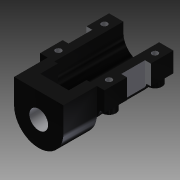
# Autodesk Inventor part: CueHolderBottom
Saved by Autodesk Inventor 2015 (Build 190159000, 159)
## iProperties
Created: 2017-01-09
Part Number: CueHolderBottom
Material: Generic
Document SubType Name: Modeling
Designer: Ernest
Density: 1 g/cm^3
Appearance: Default
Mass: 9.52114 g
Surface Area: 51.2118 cm^2
Volume: 9.52114 cm^3
Author: Ernest
Autodesk Inventor part; units mm, degrees
ref_plane "YZ Plane" through (0, 0, 0) normal (1, 0, 0) x (0, 1, 0)
ref_plane "XZ Plane" through (0, 0, 0) normal (0, 1, 0) x (-1, 0, 0)
ref_plane "XY Plane" through (0, 0, 0) normal (0, 0, 1) x (1, 0, 0)
sketch "Sketch1" plane through (0, 0, 0) normal (0, 0, 1) x (1, 0, 0)
  circle A0 centre (0, 0) radius 3
  circle A1 centre (51.029, 0) radius 3
  circle A2 centre (0, 0) radius 6
  circle A3 centre (51.029, 0) radius 6
  line L0 (11.2237, 0) -> (17.9507, 0)
  line L1 (33.0783, 0) -> (39.8053, 0)
  line L2 (16.4475, -5) -> (16.4475, 0)
  line L3 (34.5815, -5) -> (34.5815, 0)
  line L4 (18.5272, 44.067) -> (39.0012, 44.067) construction
  line L5 (8.015, 33.5) -> (43.014, 33.5) construction
  line L6 (43.014, 33.5) -> (43.014, 15.5) construction
  line L7 (43.014, 15.5) -> (8.015, 15.5) construction
  line L8 (8.015, 15.5) -> (8.015, 33.5) construction
  line L9 (14.489, 24.5) -> (38.452, 24.5) construction
  line L10 (22.5145, 29) -> (28.5145, 29)
  line L11 (28.5145, 29) -> (28.5145, 20)
  line L12 (28.5145, 20) -> (22.5145, 20)
  line L13 (22.5145, 20) -> (22.5145, 29)
  line L14 (25.5145, 33.5) -> (25.5145, 15.5) construction
  line L15 (4.5826, 10) -> (46.4464, 10)
  line L16 (-13, 10) -> (-13, -10)
  line L17 (64.029, 10) -> (64.029, -10)
  line L18 (-13, 10) -> (-4.5826, 10)
  line L19 (-13, -10) -> (-4.5826, -10)
  line L20 (64.029, 10) -> (55.6116, 10)
  line L21 (64.029, -10) -> (55.6116, -10)
  arc A4 (11.8571, -10) -> (39.1719, -10) centre (25.5145, -5) ccw
  arc A5 (16.4475, -5) -> (34.5815, -5) centre (25.5145, -5) ccw
  arc A6 (33.0783, 0) -> (17.9507, 0) centre (25.5145, -5) ccw
  line L22 (46.4464, -10) -> (39.1719, -10)
  line L23 (4.5826, -10) -> (11.8571, -10)
  line L24 (11.2237, 0) -> (11.2237, -10)
  line L25 (39.8053, 0) -> (39.8053, -10)
  arc A7 (46.4464, -10) -> (55.6116, -10) centre (51.029, 0) ccw
  arc A8 (55.6116, 10) -> (46.4464, 10) centre (51.029, 0) ccw
  arc A9 (4.5826, 10) -> (-4.5826, 10) centre (0, 0) ccw
  arc A10 (-4.5826, -10) -> (4.5826, -10) centre (0, 0) ccw
  line L26 (30.5145, 26.5) -> (17.5145, 26.5)
  line L27 (17.5145, 26.5) -> (17.5145, 10)
  line L28 (17.5145, 10) -> (30.5145, 10)
  line L29 (30.5145, 10) -> (30.5145, 26.5)
  line L30 (-13, 0) -> (64.029, 0)
  point P0 (6, 0)
  point P1 (45.029, 0)
  dimension "d144" = 12
  dimension "d146" = 12
  dimension "d143" = 6
  dimension "d145" = 6
  dimension "d147" = 51.029
  dimension "d148" = 77.029
  dimension "d149" = 20
  dimension "d150" = 11
  dimension "d151" = 11
  dimension "d152" = 11
  dimension "d153" = 11
  dimension "d154" = 9.067
  dimension "d155" = 25.5145
  dimension "d156" = 5
  dimension "d157" = 9.067
  dimension "d158" = 13
  dimension "d159" = 14.5439
  dimension "d160" = 11.2238
  dimension "d161" = 11.2238
  constraints: 62 end point, 14 point on circle, 11 point on line, 9 centre point, 9 horizontal, 7 parallel, 7 perpendicular, 6 coincident, 6 midpoint, 5 collinear, 2 horizontal alignment, 2 tangent, 2 vertical, 4 other
  measures "d143" diameter of A0
  measures "d145" diameter of A1
  measures "d147" distance of A1.centre point (0, 0)
  measures "d148" distance of L30.end L30.start
  measures "d149" distance between parallel lines of L18 L19
  measures "d150" radius of A9
  measures "d151" radius of A10
  measures "d152" radius of A8
  measures "d153" radius of A7
  measures "d154" radius of A6
  measures "d155" horizontal distance of point (0, 0) A5.centre
  measures "d156" vertical distance of point (0, 0) A5.centre
  measures "d157" radius of A5
  measures "d158" distance from line of point (0, 0) L16
  measures "d159" radius of A4
  measures "d160" distance from line of point (0, 0) L24
  measures "d161" distance from line of A1.centre L25
extrude "Extrusion1" add sketch "Sketch1" along normal blind 35 contours L30 A0 | L30 A2 A0 | A0 L30 A2 | A0 L30 | L30 L24 L23 A10 L19 L16 A2 | A2 L30 L16 L18 A9 L15 A8 L20 L17 A3 L1 A6 L0 | L0 L2 A5 L3 L1 L25 L22 A4 L23 L24 | L0 L30 L1 L3 A5 L2 | A6 L30 | L25 L30 A3 L17 L21 A7 L22 | L27 L26 L13 L12 L11 L29 L15 | L30 A1 A3 | A3 L30 A1 | L26 L11 L12 L13 | L30 A1 | A1 L30
extrude "Extrusion2" cut sketch "Sketch1" along normal blind 35 contours L30 A0 | L30 A2 A0 | A0 L30 A2 | A0 L30 | L0 L30 L1 L3 A5 L2 | A6 L30 | L30 A1 A3 | A3 L30 A1 | L30 A1 | A1 L30
ref_plane "Work Plane1" through (55.6116, 0, 0) normal (0, 1, 0) x (1, 0, 0)
sketch "Sketch2" plane through (55.6116, 0, 0) normal (0, 1, 0) x (1, 0, 0)
  line L0 (-61.6116, -35) -> (-61.6116, 0)
  line L1 (-68.6116, 0) -> (-61.6116, 0)
  line L2 (-68.6116, -35) -> (-68.6116, 0)
  line L3 (-68.6116, -35) -> (-61.6116, -35)
  line L4 (1.4174, 0) -> (1.4174, -35)
  line L5 (1.4174, -35) -> (8.4174, -35)
  line L6 (8.4174, -35) -> (8.4174, 0)
  line L7 (1.4174, 0) -> (8.4174, 0)
  line L8 (-60.0873, -35) -> (-68.6116, -35)
  line L9 (-68.6116, 0) -> (-67.4686, 0)
  line L10 (-67.4686, 0) -> (-67.4686, -35)
  line L11 (-67.4686, -35) -> (-68.6116, -35)
  line L12 (-68.6116, -35) -> (-68.6116, 0)
  line L13 (1.4174, -35) -> (8.4174, -35)
  line L14 (8.4174, 0) -> (7.2744, 0)
  line L15 (7.2744, 0) -> (7.2744, -35)
  line L16 (7.2744, -35) -> (8.4174, -35)
  line L17 (8.4174, -35) -> (8.4174, 0)
  circle A0 centre (-64.5401, -17.5) radius 1.5
  circle A1 centre (4.3459, -17.5) radius 1.5
  circle A2 centre (-46.6831, -17.5) radius 1.5
  circle A3 centre (-13.5111, -17.5) radius 1.5
  line L18 (-49.6116, 0) -> (-49.6116, -35)
  line L19 (-49.6116, -35) -> (-37.6608, -35)
  line L20 (-37.6608, -35) -> (-37.6608, 0)
  line L21 (-49.6116, 0) -> (-37.6608, 0)
  line L22 (-10.5826, -35) -> (-10.5826, 0)
  line L23 (-22.5333, 0) -> (-10.5826, 0)
  line L24 (-22.5333, -35) -> (-22.5333, 0)
  line L25 (-22.5333, -35) -> (-10.5826, -35)
  circle A4 centre (-42.9266, -5.833) radius 1.5
  circle A5 centre (-42.9266, -29.167) radius 1.5
  circle A6 centre (-17.2676, -5.833) radius 1.5
  circle A7 centre (-17.2676, -29.167) radius 1.5
  line L26 (1.4174, -0.0847) -> (1.4174, -35.0847)
  line L27 (-49.6116, -0.0847) -> (-49.6116, -35.0847)
  line L28 (-49.6116, -35) -> (-61.6116, -35) projected
  line L29 (-61.6116, 0) -> (-49.6116, 0) projected
  line L30 (1.4174, -35) -> (-10.5826, -35) projected
  line L31 (-10.5826, 0) -> (1.4174, 0) projected
  line L32 (-68.6116, 0) -> (-68.6116, -35) projected
  line L33 (-68.6116, 0) -> (-68.6116, -35) projected
  line L34 (-10.5826, 0) -> (1.4174, 0) projected
  line L35 (-61.6116, 0) -> (-49.6116, 0) projected
  line L36 (-25.0971, 0) -> (-38.0971, 0) projected
  line L37 (-9.1652, 0) -> (-25.0971, 0) projected
  line L38 (0, 0) -> (-9.1652, 0) projected
  line L39 (8.4174, 0) -> (0, 0) projected
  line L40 (0, 0) -> (8.4174, 0) projected
  line L41 (-9.1652, 0) -> (0, 0) projected
  line L42 (-16.4396, 0) -> (-9.1652, 0) projected
  line L43 (-43.7545, 0) -> (-16.4396, 0) projected
  line L44 (-51.029, 0) -> (-43.7545, 0) projected
  line L45 (-60.1942, 0) -> (-51.029, 0) projected
  line L46 (-68.6116, 0) -> (-60.1942, 0) projected
  line L47 (-60.1942, 0) -> (-68.6116, 0) projected
  line L48 (-51.029, 0) -> (-60.1942, 0) projected
  line L49 (-38.0971, 0) -> (-51.029, 0) projected
  line L50 (8.4174, 0) -> (8.4174, -35) projected
  line L51 (8.4174, 0) -> (8.4174, -35) projected
  line L52 (1.4174, -35) -> (-10.5826, -35) projected
  line L53 (-49.6116, -35) -> (-61.6116, -35) projected
  line L54 (-16.4396, -35) -> (-9.1652, -35) projected
  line L55 (-9.1652, -35) -> (0, -35) projected
  line L56 (0, -35) -> (8.4174, -35) projected
  line L57 (8.4174, -35) -> (0, -35) projected
  line L58 (0, -35) -> (-9.1652, -35) projected
  line L59 (-9.1652, -35) -> (-25.0971, -35) projected
  line L60 (-25.0971, -35) -> (-38.0971, -35) projected
  line L61 (-38.0971, -35) -> (-51.029, -35) projected
  line L62 (-51.029, -35) -> (-60.1942, -35) projected
  line L63 (-60.1942, -35) -> (-68.6116, -35) projected
  line L64 (-68.6116, -35) -> (-60.1942, -35) projected
  line L65 (-60.1942, -35) -> (-51.029, -35) projected
  line L66 (-51.029, -35) -> (-43.7545, -35) projected
  line L67 (-43.7545, -35) -> (-16.4396, -35) projected
  line L68 (-68.6116, 0) -> (8.4174, 0)
  line L69 (8.4174, 0) -> (8.4174, -35)
  line L70 (8.4174, -35) -> (-68.6116, -35)
  line L71 (-68.6116, -35) -> (-68.6116, 0)
  point P0 (-55.5011, -35.0847)
  dimension "d50" = 3
  dimension "d52" = 3
  dimension "d58" = 35
  dimension "d59" = 17.5
  dimension "d60" = 17.5
  dimension "d61" = 3
  dimension "d62" = 3
  dimension "d63" = 17.5
  dimension "d64" = 17.5
  dimension "d65" = 2.9285
  dimension "d66" = 2.9285
  dimension "d67" = 3
  dimension "d68" = 3
  dimension "d69" = 3
  dimension "d70" = 3
  dimension "d71" = 5.833
  dimension "d72" = 5.833
  dimension "d73" = 5.833
  dimension "d74" = 5.833
  dimension "d75" = 6.685
  dimension "d76" = 6.685
  dimension "d77" = 6.685
  dimension "d78" = 6.685
  dimension "d139" = 5.857
  dimension "d140" = 5.857
  dimension "d141" = 2.9285
  dimension "d142" = 2.9285
  dimension "d166" = 1.143
  dimension "d168" = 12
  dimension "d169" = 12
  dimension "d170" = 15.1275
  dimension "d171" = 11.9507
  dimension "d172" = 11.9507
  dimension "d173" = 1.143
  constraints: 64 end point, 15 collinear, 8 centre point, 6 parallel, 3 horizontal, 3 perpendicular, 2 point on line
  measures "d50" diameter of A0
  measures "d52" diameter of A1
  measures "d58" distance of L0.start L0.end
  measures "d59" distance from line of L8 A0.centre
  measures "d60" distance from line of L5 A1.centre
  measures "d61" diameter of A2
  measures "d62" diameter of A3
  measures "d63" distance from line of L8 A2.centre
  measures "d64" distance from line of L13 A3.centre
  measures "d65" distance from line of L18 A2.centre
  measures "d66" distance from line of L22 A3.centre
  measures "d67" diameter of A4
  measures "d68" diameter of A5
  measures "d69" diameter of A6
  measures "d70" diameter of A7
  measures "d71" distance from line of L21 A4.centre
  measures "d72" distance from line of L19 A5.centre
  measures "d73" distance from line of L23 A6.centre
  measures "d74" distance from line of L25 A7.centre
  measures "d75" distance from line of L18 A4.centre
  measures "d76" distance from line of L18 A5.centre
  measures "d77" distance from line of L22 A6.centre
  measures "d78" distance from line of L22 A7.centre
  measures "d139" distance between parallel lines of L0 L10
  measures "d140" distance between parallel lines of L15 L4
  measures "d141" distance from line of L0 A0.centre
  measures "d142" distance from line of L4 A1.centre
  measures "d166" distance between parallel lines of L15 L17
  measures "d168" distance between parallel lines of L18 L0
  measures "d169" distance between parallel lines of L26 L22
  measures "d170" distance between parallel lines of L24 L20
  measures "d171" distance of L18.start L20.end
  measures "d172" distance of L23.start L22.end
  measures "d173" distance between parallel lines of L2 L10
extrude "Extrusion3" cut sketch "Sketch2" along normal mid plane 35 contours L3 L2 L1 L10 | L7 L6 L5 L15 | A0 | A1 | A2 | A3 | A4 | A5 | A6 | A7
sketch "Sketch3" plane through (30.5145, 10, 0) normal (1, 0, 0) x (0, 0, -1)
  line L0 (-35, 0) -> (-35, 16.5) projected
  line L1 (-35, 14.5) -> (0, 14.5) construction
  line L2 (0, 0) -> (0, 16.5) projected
  line L3 (0, 0) -> (0, 16.5) projected
  line L4 (0, 16.5) -> (-35, 16.5) projected
  line L5 (-35, 0) -> (-35, 16.5) projected
  line L6 (0, 0) -> (-35, 0) projected
  line L7 (-35, 19) -> (0, 19)
  line L8 (0, 19) -> (0, 10)
  line L9 (0, 10) -> (-35, 10)
  line L10 (-35, 10) -> (-35, 19)
  line L11 (-35, 10) -> (0, 10)
  line L12 (0, 10) -> (0, 8.4)
  line L13 (-32.5098, 8.4) -> (-34.5098, 8.4)
  line L14 (-35, 8.4) -> (-35, 10)
  arc A0 (-35, 9.054) -> (-35, 9.746) centre (-34.5098, 9.4) ccw
  circle A1 centre (-32.5098, 9.4) radius 0.6
  line L15 (-33.7098, 9.2) -> (-33.3098, 9.2)
  arc A2 (-33.9098, 9.4) -> (-33.7098, 9.2) centre (-33.7098, 9.4) ccw
  arc A3 (-33.3098, 9.2) -> (-33.1098, 9.4) centre (-33.3098, 9.4) ccw
  arc A4 (-35, 9.746) -> (-35, 9.054) centre (-34.5098, 9.4) ccw
  line L16 (-34.5098, 8.8) -> (-34.5098, 8.4)
  line L17 (-32.5098, 8.8) -> (-32.5098, 8.4)
  point P0 (0, -10)
  point P1 (-35, 9.2)
  point P2 (0, 9.2)
  point P3 (-33.9098, 9.4)
  point P4 (-33.1098, 9.4)
  dimension "d83" = 2
  dimension "d84" = 9
  dimension "d85" = 4.5
  dimension "d86" = 1.6
  dimension "d87" = 1.2
  dimension "d88" = 1.2
  dimension "d89" = 2
  dimension "d90" = 0.8
  dimension "d91" = 0.2
  constraints: 24 end point, 12 point on circle, 8 point on line, 5 centre point, 5 horizontal, 5 perpendicular, 4 parallel, 4 tangent, 2 coincident, 2 midpoint, 1 equal radius, 8 other
  measures "d83" distance between parallel lines of L1 L4
  measures "d84" distance between parallel lines of L9 L7
  measures "d85" distance between parallel lines of L1 L7
  measures "d86" distance between parallel lines of L11 L13
  measures "d87" diameter of A0
  measures "d88" diameter of A1
  measures "d89" distance of A1.centre A0.centre
  measures "d90" distance between parallel lines of L15 L13
  measures "d91" radius of A2
extrude "Extrusion4" cut sketch "Sketch3" against normal blind 7 contours L0 A0 | A0 A2 L15 A3 A1 L17 L13 L16 | A1
pattern_linear "Rectangular Pattern1" count 18 spacing 2 along (0, 0, -1) count 2 spacing 2 along (0, 0, 1) of "Extrusion4"
sketch "Sketch4" plane through (0, 0, 35) normal (0, 0, 1) x (1, 0, 0)
  line L0 (23.5145, 18.4) -> (23.5145, 19.746) projected
  line L1 (23.5145, 19.746) -> (30.5145, 19.746) projected
  line L2 (30.5145, 19.746) -> (30.5145, 26.5) projected
  line L3 (30.5145, 26.5) -> (17.5145, 26.5) projected
  line L4 (17.5145, 26.5) -> (17.5145, 10) projected
  line L5 (17.5145, 10) -> (4.5826, 10) projected
  arc A0 (4.5826, 10) -> (-4.5826, 10) centre (0, 0) ccw projected
  line L6 (-4.5826, 10) -> (-13, 10) projected
  line L7 (64.029, 10) -> (55.6116, 10) projected
  arc A1 (55.6116, 10) -> (46.4464, 10) centre (51.029, 0) ccw projected
  line L8 (46.4464, 10) -> (30.5145, 10) projected
  line L9 (30.5145, 10) -> (30.5145, 18.4) projected
  line L10 (30.5145, 18.4) -> (23.5145, 18.4) projected
  line L11 (17.5145, 10) -> (12.5145, 10)
  line L12 (12.5145, 10) -> (12.5145, 18)
  line L13 (12.5145, 18) -> (17.5145, 18)
  line L14 (17.5145, 18) -> (17.5145, 10)
  line L15 (30.5145, 10) -> (35.5145, 10)
  line L16 (35.5145, 10) -> (35.5145, 18)
  line L17 (35.5145, 18) -> (30.5145, 18)
  line L18 (30.5145, 18) -> (30.5145, 10)
  circle A2 centre (0, 0) radius 6 projected
  circle A3 centre (51.029, 0) radius 6 projected
  line L19 (-13, -10) -> (-4.5826, -10) projected
  arc A4 (-4.5826, -10) -> (4.5826, -10) centre (0, 0) ccw projected
  line L20 (4.5826, -10) -> (11.8571, -10) projected
  arc A5 (11.8571, -10) -> (39.1719, -10) centre (25.5145, -5) ccw projected
  line L21 (39.1719, -10) -> (46.4464, -10) projected
  arc A6 (46.4464, -10) -> (55.6116, -10) centre (51.029, 0) ccw projected
  line L22 (55.6116, -10) -> (64.029, -10) projected
  line L23 (-13, 10) -> (-13, -10) projected
  line L24 (64.029, -10) -> (64.029, 10) projected
  dimension "d100" = 8
  dimension "d101" = 5
  dimension "d106" = 5
  dimension "d107" = 8
  constraints: 16 end point, 4 parallel, 2 horizontal, 2 perpendicular
  measures "d100" distance of L11.end L12.end
  measures "d101" distance of L12.end L13.end
  measures "d106" distance of L17.end L16.end
  measures "d107" distance of L16.end L15.end
extrude "Extrusion5" add sketch "Sketch4" against normal blind 26.25 contours L17 L16 L8 L9 | L4 L5 L12 L13
extrude "Extrusion6" cut sketch "Sketch4" against normal blind 8.75 contours L17 L16 L8 L9 | L4 L5 L12 L13
sketch "Sketch5" plane through (17.5145, 26.5, 0) normal (0, 1, 0) x (1, 0, 0)
  arc A0 (0, -26.25) -> (0, -23.75) centre (0, -25) ccw
  line L0 (-5, -26.25) -> (0, -26.25) projected
  line L1 (-5, -8.75) -> (0, -8.75) projected
  arc A1 (0, -21.25) -> (0, -23.75) centre (0, -22.5) ccw
  arc A2 (0, -21.25) -> (0, -18.75) centre (0, -20) ccw
  arc A3 (0, -16.25) -> (0, -18.75) centre (0, -17.5) ccw
  arc A4 (0, -16.25) -> (0, -13.75) centre (0, -15) ccw
  arc A5 (0, -11.25) -> (0, -13.75) centre (0, -12.5) ccw
  arc A6 (0, -11.25) -> (0, -8.75) centre (0, -10) ccw
  arc A7 (13, -23.75) -> (13, -26.25) centre (13, -25) ccw
  line L2 (13, -26.25) -> (18, -26.25) projected
  arc A8 (13, -23.75) -> (13, -21.25) centre (13, -22.5) ccw
  arc A9 (13, -18.75) -> (13, -21.25) centre (13, -20) ccw
  arc A10 (13, -18.75) -> (13, -16.25) centre (13, -17.5) ccw
  arc A11 (13, -13.75) -> (13, -16.25) centre (13, -15) ccw
  arc A12 (13, -13.75) -> (13, -11.25) centre (13, -12.5) ccw
  arc A13 (13, -8.75) -> (13, -11.25) centre (13, -10) ccw
  line L3 (-29.291, -35) -> (0, -35)
  line L4 (0, 0) -> (-29.291, 0)
  line L5 (-29.291, 0) -> (-29.291, -35)
  line L6 (45.3715, -35) -> (13, -35)
  line L7 (13, 0) -> (45.3715, 0)
  line L8 (45.3715, 0) -> (45.3715, -35)
  line L9 (-5, -26.25) -> (0, -26.25)
  line L10 (0, -8.75) -> (-5, -8.75)
  line L11 (-5, -8.75) -> (-5, -26.25)
  line L12 (18, -26.25) -> (13, -26.25)
  line L13 (13, -8.75) -> (18, -8.75)
  line L14 (18, -8.75) -> (18, -26.25)
  line L15 (0, -8.75) -> (0, 0)
  line L16 (0, -35) -> (0, -26.25)
  line L17 (13, -35) -> (13, -26.25)
  line L18 (13, -8.75) -> (13, 0)
  line L19 (0, -35) -> (13, -35)
  line L20 (0, 0) -> (13, 0)
  dimension "d108" = 2.5
  dimension "d109" = 17.5
  dimension "d110" = 2.5
  dimension "d111" = 2.5
  dimension "d112" = 2.5
  dimension "d113" = 2.5
  dimension "d114" = 2.5
  dimension "d115" = 2.5
  dimension "d116" = 2.5
  dimension "d117" = 2.5
  dimension "d118" = 2.5
  dimension "d119" = 2.5
  dimension "d120" = 2.5
  dimension "d121" = 2.5
  dimension "d122" = 2.5
  dimension "d162" = 5
  dimension "d163" = 5
  dimension "d164" = 13
  dimension "d165" = 74.6625
  constraints: 37 end point, 28 point on circle, 14 centre point, 13 tangent, 6 equal length, 5 horizontal, 1 point on line
  measures "d108" diameter of A0
  measures "d109" distance between parallel lines of L1 L0
  measures "d110" diameter of A1
  measures "d111" diameter of A2
  measures "d112" diameter of A3
  measures "d113" diameter of A4
  measures "d114" diameter of A5
  measures "d115" diameter of A6
  measures "d116" diameter of A7
  measures "d117" diameter of A8
  measures "d118" diameter of A9
  measures "d119" diameter of A10
  measures "d120" diameter of A11
  measures "d121" diameter of A12
  measures "d122" diameter of A13
  measures "d162" distance between parallel lines of L16 L11
  measures "d163" distance between parallel lines of L17 L14
  measures "d164" distance between parallel lines of L18 L15
  measures "d165" distance between parallel lines of L8 L5
extrude "Extrusion7" cut sketch "Sketch5" against normal blind 16.5 contours A0 A1 A2 A3 A4 A5 A6 L15 L20 L18 A13 A12 A11 A10 A9 A8 A7 L17 L19 L16
sketch "Sketch6" plane through (17.5145, 26.5, 25) normal (0, 1, 0) x (1, 0, 0)
  line L0 (-2.8394, -2.9296) -> (15.1567, -2.9296)
  line L1 (15.1567, -2.9296) -> (15.1567, 18.0113)
  line L2 (15.1567, 18.0113) -> (-2.8394, 18.0113)
  line L3 (-2.8394, 18.0113) -> (-2.8394, -2.9296)
  point P0 (-17.5145, 25)
  constraints: 8 end point, 2 parallel, 1 horizontal, 1 perpendicular
extrude "Extrusion8" cut sketch "Sketch6" against normal blind 8.5
sketch "Sketch7" plane through (35.5145, 10, 8.75) normal (1, 0, 0) x (0, 0, -1)
  line L0 (-17.5, 8) -> (-17.5, 0) projected
  line L1 (0, 0) -> (-17.5, 0) projected
  line L2 (0, 8) -> (0, 0) projected
  line L3 (-17.5, 8) -> (0, 8) projected
  line L4 (-10.25, 0) -> (-7.25, 0) projected
  line L5 (1.417, 0) -> (4.417, 0) projected
  circle A0 centre (-13.125, 4) radius 1.5
  circle A1 centre (-4.375, 4) radius 1.5
  line L6 (-8.75, 8) -> (-8.75, 0)
  line L7 (-17.5, 0) -> (0, 0) projected
  point P0 (8.75, -10)
  point P1 (-7.25, -10)
  point P2 (-10.25, -10)
  point P3 (-18.917, -10)
  point P4 (-21.917, -10)
  dimension "d127" = 3
  dimension "d128" = 3
  dimension "d129" = 8
  dimension "d130" = 17.5
  dimension "d131" = 8.75
  dimension "d132" = 4
  dimension "d133" = 4
  dimension "d134" = 4.375
  dimension "d135" = 4.375
  constraints: 2 centre point, 2 end point, 2 midpoint, 1 vertical
  measures "d127" diameter of A0
  measures "d128" diameter of A1
  measures "d129" distance of L0.start L0.end
  measures "d130" distance of L0.start L2.start
  measures "d131" distance between parallel lines of L0 L6
  measures "d132" distance from line of L3 A0.centre
  measures "d133" distance from line of L1 A1.centre
  measures "d134" distance from line of L0 A0.centre
  measures "d135" distance from line of L2 A1.centre
extrude "Extrusion9" cut sketch "Sketch7" against normal blind 25.75 contours A0 | A1
sketch "Sketch8" plane through (39.1719, -10, 0) normal (0, -1, 0) x (1, 0, 0)
  spline S0 degree 5 poles (0, 4.5822) (-0.1104, 4.5091) (-0.2304, 4.4472) (-0.3605, 4.3972) (-0.5007, 4.3614) (-0.796, 4.3262) (-0.9501, 4.3258) (-1.1137, 4.3457) (-1.2845, 4.3916) (-1.5743, 4.5255) (-1.6926, 4.5954) (-1.8098, 4.6839) (-1.9216, 4.7931) (-2.1281, 5.0647) (-2.2209, 5.2289) (-2.2923, 5.4191) (-2.3279, 5.6262) (-2.3279, 5.996) (-2.3055, 6.1592) (-2.2618, 6.314) (-2.2005, 6.4555) (-2.0783, 6.6675) (-2.0237, 6.746) (-1.965, 6.8175) (-1.9034, 6.8822) (-1.7429, 7.0289) (-1.6416, 7.102) (-1.5389, 7.1611) (-1.4367, 7.2081) (-1.0141, 7.3602) (-0.7042, 7.3683) (-0.4373, 7.3138) (-0.2033, 7.2184) (0, 7.0838) knots 0 0 0 0 0 0 0.150257 0.150257 0.150257 0.150257 0.296295 0.296295 0.296295 0.296295 0.395447 0.395447 0.395447 0.395447 0.50046 0.50046 0.50046 0.50046 0.583231 0.583231 0.583231 0.583231 0.63924 0.63924 0.63924 0.63924 0.725202 0.725202 0.725202 0.725202 1 1 1 1 1 1 projected
  arc A0 (0, 4.5822) -> (0, 7.0838) centre (-0.8279, 5.833) ccw projected
  circle A1 centre (-0.8279, 5.833) radius 1.5 projected
  spline S1 degree 5 poles (0, 27.9162) (-0.1104, 27.8431) (-0.2304, 27.7812) (-0.3605, 27.7312) (-0.5007, 27.6954) (-0.796, 27.6602) (-0.9501, 27.6598) (-1.1137, 27.6797) (-1.2845, 27.7256) (-1.5743, 27.8595) (-1.6926, 27.9294) (-1.8098, 28.0179) (-1.9216, 28.1271) (-2.1281, 28.3987) (-2.2209, 28.5629) (-2.2923, 28.7531) (-2.3279, 28.9602) (-2.3279, 29.33) (-2.3055, 29.4932) (-2.2618, 29.648) (-2.2005, 29.7895) (-2.0783, 30.0015) (-2.0237, 30.08) (-1.965, 30.1515) (-1.9034, 30.2162) (-1.7429, 30.3629) (-1.6416, 30.436) (-1.5389, 30.4951) (-1.4367, 30.5421) (-1.0141, 30.6942) (-0.7042, 30.7023) (-0.4373, 30.6478) (-0.2033, 30.5524) (0, 30.4178) knots 0 0 0 0 0 0 0.150257 0.150257 0.150257 0.150257 0.296295 0.296295 0.296295 0.296295 0.395447 0.395447 0.395447 0.395447 0.50046 0.50046 0.50046 0.50046 0.583231 0.583231 0.583231 0.583231 0.63924 0.63924 0.63924 0.63924 0.725202 0.725202 0.725202 0.725202 1 1 1 1 1 1 projected
  arc A2 (0, 27.9162) -> (0, 30.4178) centre (-0.8279, 29.167) ccw projected
  circle A3 centre (-0.8279, 29.167) radius 1.5 projected
  spline S2 degree 8 poles (-27.3149, 30.4178) (-27.2459, 30.4635) (-27.1734, 30.5052) (-27.0975, 30.5428) (-27.018, 30.576) (-26.9349, 30.6044) (-26.8483, 30.6277) (-26.7581, 30.6453) (-26.5735, 30.6673) (-26.4794, 30.6721) (-26.3822, 30.6702) (-26.2818, 30.6609) (-26.1786, 30.6433) (-26.073, 30.6163) (-25.9657, 30.5785) (-25.7845, 30.4948) (-25.7108, 30.4553) (-25.6372, 30.4097) (-25.5641, 30.3575) (-25.4923, 30.2984) (-25.4225, 30.2318) (-25.3557, 30.1575) (-25.2689, 30.0433) (-25.2454, 30.0104) (-25.2226, 29.9763) (-25.2006, 29.9411) (-25.1794, 29.9047) (-25.1592, 29.8672) (-25.1401, 29.8287) (-25.0904, 29.7196) (-25.0387, 29.5867) (-25, 29.4439) (-24.9772, 29.294) (-24.9719, 29.1407) (-24.9851, 28.9871) (-25.0151, 28.8414) (-25.059, 28.703) (-25.0928, 28.6126) (-25.1046, 28.5832) (-25.117, 28.5543) (-25.13, 28.526) (-25.1436, 28.4981) (-25.1577, 28.4709) (-25.1722, 28.4442) (-25.2181, 28.3646) (-25.2508, 28.3136) (-25.2853, 28.2651) (-25.3211, 28.2191) (-25.3582, 28.1756) (-25.3963, 28.1346) (-25.4353, 28.0961) (-25.5355, 28.0044) (-25.5978, 27.9545) (-25.661, 27.9099) (-25.7247, 27.8703) (-25.7886, 27.8354) (-25.8524, 27.8048) (-25.9159, 27.7783) (-26.18, 27.6832) (-26.3771, 27.6493) (-26.564, 27.6458) (-26.7386, 27.6664) (-26.9004, 27.7061) (-27.0499, 27.762) (-27.1878, 27.8321) (-27.3149, 27.9162) knots 0 0 0 0 0 0 0 0 0 0.150381 0.150381 0.150381 0.150381 0.150381 0.150381 0.150381 0.29654 0.29654 0.29654 0.29654 0.29654 0.29654 0.29654 0.395774 0.395774 0.395774 0.395774 0.395774 0.395774 0.395774 0.433966 0.433966 0.433966 0.433966 0.433966 0.433966 0.433966 0.500813 0.556206 0.556206 0.556206 0.556206 0.556206 0.556206 0.556206 0.583535 0.583535 0.583535 0.583535 0.583535 0.583535 0.583535 0.639503 0.639503 0.639503 0.639503 0.639503 0.639503 0.639503 0.725403 0.725403 0.725403 0.725403 0.725403 0.725403 0.725403 1 1 1 1 1 1 1 1 1 projected
  arc A4 (-27.3149, 30.4178) -> (-27.3149, 27.9162) centre (-26.4869, 29.167) ccw projected
  circle A5 centre (-26.4869, 29.167) radius 1.5 projected
  spline S3 degree 8 poles (-27.3149, 7.0838) (-27.2459, 7.1295) (-27.1734, 7.1712) (-27.0975, 7.2088) (-27.018, 7.242) (-26.9349, 7.2704) (-26.8483, 7.2937) (-26.7581, 7.3113) (-26.5735, 7.3333) (-26.4794, 7.3381) (-26.3822, 7.3362) (-26.2818, 7.3269) (-26.1786, 7.3093) (-26.073, 7.2823) (-25.9657, 7.2445) (-25.7845, 7.1608) (-25.7108, 7.1213) (-25.6372, 7.0757) (-25.5641, 7.0235) (-25.4923, 6.9644) (-25.4225, 6.8978) (-25.3557, 6.8235) (-25.2689, 6.7093) (-25.2454, 6.6764) (-25.2226, 6.6423) (-25.2006, 6.6071) (-25.1794, 6.5707) (-25.1592, 6.5332) (-25.1401, 6.4947) (-25.0904, 6.3856) (-25.0387, 6.2527) (-25, 6.1099) (-24.9772, 5.96) (-24.9719, 5.8067) (-24.9851, 5.6531) (-25.0151, 5.5074) (-25.059, 5.369) (-25.0928, 5.2786) (-25.1046, 5.2492) (-25.117, 5.2203) (-25.13, 5.192) (-25.1436, 5.1641) (-25.1577, 5.1369) (-25.1722, 5.1102) (-25.2181, 5.0306) (-25.2508, 4.9796) (-25.2853, 4.9311) (-25.3211, 4.8851) (-25.3582, 4.8416) (-25.3963, 4.8006) (-25.4353, 4.7621) (-25.5355, 4.6704) (-25.5978, 4.6205) (-25.661, 4.5759) (-25.7247, 4.5363) (-25.7886, 4.5014) (-25.8524, 4.4708) (-25.9159, 4.4443) (-26.18, 4.3492) (-26.3771, 4.3153) (-26.564, 4.3118) (-26.7386, 4.3324) (-26.9004, 4.3721) (-27.0499, 4.428) (-27.1878, 4.4981) (-27.3149, 4.5822) knots 0 0 0 0 0 0 0 0 0 0.150381 0.150381 0.150381 0.150381 0.150381 0.150381 0.150381 0.29654 0.29654 0.29654 0.29654 0.29654 0.29654 0.29654 0.395774 0.395774 0.395774 0.395774 0.395774 0.395774 0.395774 0.433966 0.433966 0.433966 0.433966 0.433966 0.433966 0.433966 0.500813 0.556206 0.556206 0.556206 0.556206 0.556206 0.556206 0.556206 0.583535 0.583535 0.583535 0.583535 0.583535 0.583535 0.583535 0.639503 0.639503 0.639503 0.639503 0.639503 0.639503 0.639503 0.725403 0.725403 0.725403 0.725403 0.725403 0.725403 0.725403 1 1 1 1 1 1 1 1 1 projected
  arc A6 (-27.3149, 7.0838) -> (-27.3149, 4.5822) centre (-26.4869, 5.833) ccw projected
  circle A7 centre (-26.4869, 5.833) radius 1.5 projected
  circle A8 centre (-0.8279, 5.833) radius 3.5
  circle A9 centre (-26.4869, 5.833) radius 3.5
  circle A10 centre (-26.4869, 29.167) radius 3.5
  circle A11 centre (-0.8279, 29.167) radius 3.5
  point P0 (-39.1719, 0)
  dimension "d174" = 7
  dimension "d175" = 7
  dimension "d176" = 7
  dimension "d177" = 7
  constraints: 4 centre point, 4 coincident, 4 vertical alignment
  measures "d174" diameter of A8
  measures "d175" diameter of A9
  measures "d176" diameter of A10
  measures "d177" diameter of A11
extrude "Extrusion10" cut sketch "Sketch8" along normal blind 16.5
extrude "Extrusion11" add sketch "Sketch8" along normal blind 3
sketch "Sketch9" plane through (0, 0, 0) normal (0, 0, -1) x (-1, 0, 0)
  line L0 (-62.8862, 10) -> (11.857, 10)
  line L1 (11.857, 10) -> (11.857, 35.2679)
  line L2 (11.857, 35.2679) -> (-62.8862, 35.2679)
  line L3 (-62.8862, 35.2679) -> (-62.8862, 10)
  point P0 (0, 0)
  constraints: 8 end point, 2 parallel, 1 horizontal, 1 perpendicular
extrude "Extrusion12" cut sketch "Sketch9" against normal blind 35
extrude "Extrusion13" cut sketch "Sketch1" along normal blind 35 contours L30 A0 | A0 L30 A2 | A2 L30 L16 L18 A9 L15 A8 L20 L17 A3 L1 A6 L0 | A6 L30 | A3 L30 A1 | A1 L30 picked at (0.7485, 0.6631) picked at (3.2012, 3.7952) picked at (54.2302, 3.7952) picked at (51.5971, 1.7524)
sketch "Sketch10" plane through (34.5815, 0, 0) normal (0, 1, 0) x (1, 0, 0)
  circle A0 centre (3.7625, -5.833) radius 1.5 projected
  circle A1 centre (7.519, -17.5) radius 1.5 projected
  circle A2 centre (3.7625, -29.167) radius 1.5 projected
  line L0 (10.4475, 0) -> (10.4475, -35) projected
  line L1 (0, 0) -> (10.4475, 0) projected
  line L2 (0, 0) -> (0, -35) projected
  line L3 (10.4475, -35) -> (0, -35) projected
  circle A3 centre (-25.653, -17.5) radius 1.5 projected
  circle A4 centre (-21.8965, -5.833) radius 1.5 projected
  circle A5 centre (-21.8965, -29.167) radius 1.5 projected
  line L4 (-18.134, 0) -> (-18.134, -35) projected
  line L5 (-28.5815, 0) -> (-18.134, 0) projected
  line L6 (-28.5815, -35) -> (-28.5815, 0) projected
  line L7 (-18.134, -35) -> (-28.5815, -35) projected
  line L8 (22.4475, -35) -> (22.4475, 0) projected
  line L9 (10.4475, -35) -> (0, -35) projected
  line L10 (0, 0) -> (10.4475, 0) projected
  circle A6 centre (25.376, -17.5) radius 1.5 projected
  circle A7 centre (-43.51, -17.5) radius 1.5 projected
  line L11 (-40.5815, 0) -> (-40.5815, -35) projected
  line L12 (0, 0) -> (10.4475, 0) projected
  line L13 (10.4475, -35) -> (0, -35) projected
  circle A8 centre (7.519, -17.5) radius 1.5 projected
  arc A9 (4.5904, -9.2337) -> (4.5904, -2.4323) centre (3.7625, -5.833) ccw projected
  line L14 (4.5904, 0) -> (4.5904, -2.4323) projected
  line L15 (4.5904, 0) -> (11.8649, 0) projected
  line L16 (11.8649, 0) -> (11.8649, -35) projected
  line L17 (4.5904, -35) -> (11.8649, -35) projected
  line L18 (4.5904, -32.5677) -> (4.5904, -35) projected
  arc A10 (4.5904, -32.5677) -> (4.5904, -25.7663) centre (3.7625, -29.167) ccw projected
  line L19 (4.5904, -9.2337) -> (4.5904, -25.7663) projected
  circle A11 centre (-25.653, -17.5) radius 1.5 projected
  arc A12 (-22.7244, -25.7663) -> (-22.7244, -32.5677) centre (-21.8965, -29.167) ccw projected
  line L20 (-22.7244, -32.5677) -> (-22.7244, -35) projected
  line L21 (-29.9989, -35) -> (-22.7244, -35) projected
  line L22 (-29.9989, 0) -> (-29.9989, -35) projected
  line L23 (-29.9989, 0) -> (-22.7244, 0) projected
  line L24 (-22.7244, 0) -> (-22.7244, -2.4323) projected
  arc A13 (-22.7244, -2.4323) -> (-22.7244, -9.2337) centre (-21.8965, -5.833) ccw projected
  line L25 (-22.7244, -9.2337) -> (-22.7244, -25.7663) projected
  line L26 (0, 0) -> (10.4475, 0) projected
  line L27 (7.2627, 0) -> (7.2627, -35)
  line L28 (4.5904, -35) -> (11.8649, -35) projected
  line L29 (-29.9989, -35) -> (-22.7244, -35) projected
  line L30 (-25.3965, -35) -> (-25.3965, 0)
  line L31 (-29.9989, 0) -> (-22.7244, 0) projected
  line L32 (7.2627, -35) -> (-25.3965, -35)
  line L33 (7.2627, 0) -> (-25.3965, 0)
  line L34 (4.5904, 0) -> (11.8649, 0) projected
  line L35 (4.5904, -9.2337) -> (4.5904, -25.7663) projected
  line L36 (7.2627, -23.332) -> (4.5904, -23.332)
  line L37 (4.5904, -23.332) -> (4.5904, -11.668)
  line L38 (4.5904, -11.668) -> (7.2627, -11.668)
  line L39 (7.2627, -11.668) -> (7.2627, -23.332)
  line L40 (-22.7244, -9.2337) -> (-22.7244, -25.7663) projected
  line L41 (-22.7244, -23.332) -> (-25.3965, -23.332)
  line L42 (-25.3965, -23.332) -> (-25.3965, -11.668)
  line L43 (-25.3965, -11.668) -> (-22.7244, -11.668)
  line L44 (-22.7244, -11.668) -> (-22.7244, -23.332)
  line L45 (28.3047, -35) -> (7.2627, -35)
  line L46 (7.2627, -35) -> (7.2627, 0)
  line L47 (7.2627, 0) -> (28.3047, 0)
  line L48 (28.3047, 0) -> (28.3047, -35)
  line L49 (-46.4385, -35) -> (-25.3965, -35)
  line L50 (-25.3965, -35) -> (-25.3965, 0)
  line L51 (-25.3965, 0) -> (-46.4385, 0)
  line L52 (-46.4385, 0) -> (-46.4385, -35)
  line L53 (-18.134, 0) -> (-18.134, -35) projected
  line L54 (-28.5815, 0) -> (-18.134, 0) projected
  line L55 (-28.5815, -35) -> (-28.5815, 0) projected
  line L56 (-18.134, -35) -> (-28.5815, -35) projected
  line L57 (-47.5815, 0) -> (-40.5815, 0) projected
  line L58 (-47.5815, -35) -> (-47.5815, 0) projected
  line L59 (-40.5815, -35) -> (-47.5815, -35) projected
  line L60 (22.4475, -35) -> (22.4475, 0) projected
  line L61 (29.4475, -35) -> (22.4475, -35) projected
  line L62 (29.4475, 0) -> (29.4475, -35) projected
  line L63 (22.4475, 0) -> (29.4475, 0) projected
  line L64 (10.4475, 0) -> (10.4475, -35) projected
  line L65 (0, 0) -> (0, -35) projected
  line L66 (-18.134, 0) -> (-18.134, -35) projected
  line L67 (-28.5815, 0) -> (-18.134, 0) projected
  line L68 (-28.5815, -35) -> (-28.5815, 0) projected
  line L69 (-18.134, -35) -> (-28.5815, -35) projected
  line L70 (-40.5815, 0) -> (-40.5815, -35) projected
  line L71 (-47.5815, 0) -> (-40.5815, 0) projected
  line L72 (-47.5815, -35) -> (-47.5815, 0) projected
  line L73 (-40.5815, -35) -> (-47.5815, -35) projected
  line L74 (29.4475, -35) -> (22.4475, -35) projected
  line L75 (29.4475, 0) -> (29.4475, -35) projected
  line L76 (22.4475, 0) -> (29.4475, 0) projected
  line L77 (10.4475, 0) -> (10.4475, -35) projected
  line L78 (0, 0) -> (0, -35) projected
  point P0 (-34.5815, 0)
  dimension "d186" = 11.6641
  dimension "d187" = 5.832
  dimension "d188" = 5.832
  dimension "d189" = 5.832
  dimension "d190" = 5.832
  constraints: 40 end point, 9 parallel, 8 point on line, 5 horizontal, 5 perpendicular, 1 collinear
  measures "d187" distance from line of A3.centre L41
  measures "d188" distance from line of A3.centre L43
  measures "d189" distance from line of A1.centre L36
  measures "d190" distance from line of A1.centre L38
extrude "Extrusion14" cut sketch "Sketch10" against normal blind 35 contours A1 L27 | A1 L27 L1 L0 L3 | L27 A1 | A1 L27 L36 L19 L38 | L15 L16 L17 L0 | L47 L8 L45 L16 | L47 L48 L45 L8 | L63 L62 L61 L48 | L30 A3 L7 L6 L5 | L6 L21 L22 L23 | L22 L49 L11 L51 | L43 L25 L41 L30 A3 | L11 L49 L52 L51 | L30 A3 | A3 L30 | L52 L59 L58 L57
sketch "Sketch12" plane through (0, 0, 35) normal (0, 0, 1) x (1, 0, 0)
  line L0 (9.185, 0) -> (9.185, -10) projected
  line L1 (9.185, -10) -> (11.8571, -10) projected
  arc A0 (11.8571, -10) -> (39.1719, -10) centre (25.5145, -5) ccw projected
  line L2 (39.1719, -10) -> (41.8442, -10) projected
  line L3 (41.8442, -10) -> (41.8442, 0) projected
  line L4 (41.8442, 0) -> (34.5815, 0) projected
  line L5 (34.5815, 0) -> (34.5815, -5) projected
  arc A1 (16.4475, -5) -> (34.5815, -5) centre (25.5145, -5) ccw projected
  line L6 (16.4475, -5) -> (16.4475, 0) projected
  line L7 (16.4475, 0) -> (9.185, 0) projected
  arc A2 (11.3724, 0) -> (39.6566, 0) centre (25.5145, -5) ccw
  line L8 (11.3724, 0) -> (39.6566, 0)
  line L9 (39.844, 0) -> (36.844, 0) projected
  point P0 (0, 0)
  dimension "d193" = 30
  constraints: 2 end point, 2 point on circle, 2 point on line, 1 centre point, 1 coincident, 1 collinear
  measures "d193" diameter of A2
extrude "Extrusion15" add sketch "Sketch12" against normal blind 35 contours L7 L6 A1 L5 L4 A2 L2 A0 L1 | L1 A0 L2 A2
sketch "Sketch13" plane through (16.4475, 0, 35) normal (0, 1, 0) x (1, 0, 0)
  arc A0 (-5.0751, 29.8929) -> (-5.0751, 28.4411) centre (-3.7625, 29.167) ccw projected
  line L0 (-5.0751, 28.4411) -> (-5.0751, 29.8929) projected
  line L1 (-5.0751, 11.668) -> (-5.0751, 23.332) projected
  line L2 (-5.0751, 11.668) -> (-7.2625, 11.668) projected
  line L3 (-7.2625, 11.668) -> (-7.2625, 0) projected
  line L4 (0, 0) -> (-7.2625, 0) projected
  line L5 (0, 35) -> (0, 0) projected
  line L6 (-7.2625, 35) -> (0, 35) projected
  line L7 (-7.2625, 35) -> (-7.2625, 23.332) projected
  line L8 (-7.2625, 23.332) -> (-5.0751, 23.332) projected
  line L9 (-5.0751, 5.1071) -> (-5.0751, 6.5589) projected
  arc A1 (-5.0751, 6.5589) -> (-5.0751, 5.1071) centre (-3.7625, 5.833) ccw projected
  arc A2 (23.2091, 28.4411) -> (23.2091, 29.8929) centre (21.8965, 29.167) ccw projected
  line L10 (23.2091, 28.4411) -> (23.2091, 29.8929) projected
  line L11 (18.134, 35) -> (25.3967, 35) projected
  line L12 (18.134, 35) -> (18.134, 0) projected
  line L13 (25.3967, 0) -> (18.134, 0) projected
  line L14 (25.3967, 0) -> (25.3967, 11.668) projected
  line L15 (25.3967, 11.668) -> (23.2091, 11.668) projected
  line L16 (23.2091, 11.668) -> (23.2091, 23.332) projected
  line L17 (23.2091, 23.332) -> (25.3967, 23.332) projected
  line L18 (25.3967, 23.332) -> (25.3967, 35) projected
  arc A3 (23.2091, 5.1071) -> (23.2091, 6.5589) centre (21.8965, 5.833) ccw projected
  line L19 (23.2091, 5.1071) -> (23.2091, 6.5589) projected
  line L20 (-7.2625, 23.332) -> (-4.5905, 23.332)
  line L21 (-4.5905, 23.332) -> (-4.5905, 11.668)
  line L22 (-4.5905, 11.668) -> (-7.2625, 11.668)
  line L23 (-7.2625, 11.668) -> (-7.2625, 23.332)
  line L24 (25.3967, 23.332) -> (22.7245, 23.332)
  line L25 (22.7245, 23.332) -> (22.7245, 11.668)
  line L26 (22.7245, 11.668) -> (25.3967, 11.668)
  line L27 (25.3967, 11.668) -> (25.3967, 23.332)
  point P0 (-16.4475, 35)
  dimension "d196" = 27.315
  dimension "d197" = 0.4846
  dimension "d198" = 28.2843
  constraints: 16 end point, 4 parallel, 2 horizontal, 2 perpendicular, 1 point on line
  measures "d196" distance between parallel lines of L25 L21
  measures "d197" distance between parallel lines of L21 L1
  measures "d198" distance between parallel lines of L16 L1
extrude "Extrusion16" cut sketch "Sketch13" against normal blind 35 contours L2 L23 L8 L1 | L1 L20 L21 L22 | L27 L15 L16 L17 | L16 L26 L25 L24
sketch "Sketch14" plane through (39.1719, -13, 0) normal (0, -1, 0) x (1, 0, 0)
  line L0 (-26.346, 25.6698) -> (-26.346, 27.6736) projected
  arc A0 (-27.3149, 30.4178) -> (-27.3149, 27.9162) centre (-26.4869, 29.167) ccw projected
  line L1 (-26.346, 30.6604) -> (-26.346, 32.6642) projected
  arc A1 (-26.346, 32.6642) -> (-26.346, 25.6698) centre (-26.4869, 29.167) ccw projected
  line L2 (-26.346, 7.3264) -> (-26.346, 9.3302) projected
  arc A2 (-26.346, 9.3302) -> (-26.346, 2.3358) centre (-26.4869, 5.833) ccw projected
  line L3 (-26.346, 2.3358) -> (-26.346, 4.3396) projected
  arc A3 (-27.3149, 7.0838) -> (-27.3149, 4.5822) centre (-26.4869, 5.833) ccw projected
  line L4 (-0.9689, 32.6642) -> (-0.9689, 30.6604) projected
  arc A4 (0, 27.9162) -> (0, 30.4178) centre (-0.8279, 29.167) ccw projected
  line L5 (-0.9689, 27.6736) -> (-0.9689, 25.6698) projected
  arc A5 (-0.9689, 25.6698) -> (-0.9689, 32.6642) centre (-0.8279, 29.167) ccw projected
  line L6 (-0.9689, 4.3396) -> (-0.9689, 2.3358) projected
  arc A6 (-0.9689, 2.3358) -> (-0.9689, 9.3302) centre (-0.8279, 5.833) ccw projected
  line L7 (-0.9689, 9.3302) -> (-0.9689, 7.3264) projected
  arc A7 (0, 4.5822) -> (0, 7.0838) centre (-0.8279, 5.833) ccw projected
  circle A8 centre (-26.4869, 29.167) radius 3.5
  circle A9 centre (-26.4869, 29.167) radius 1.5
  circle A10 centre (-0.8279, 29.167) radius 1.5
  circle A11 centre (-0.8279, 29.167) radius 3.5
  circle A12 centre (-26.4869, 5.833) radius 1.5
  circle A13 centre (-26.4869, 5.833) radius 3.5
  circle A14 centre (-0.8279, 5.833) radius 1.5
  circle A15 centre (-0.8279, 5.833) radius 3.5
  point P0 (-39.1719, 0)
  constraints: 8 coincident, 7 centre point, 4 concentric, 11 other
extrude "Extrusion17" cut sketch "Sketch14" along normal blind 35 contours A1 L1 A9 A0 L0 | L0 A9 L1 A8 | A12 A3 L3 A2 L2 | L2 A13 L3 A12 | A5 L5 A10 A4 L4 | L4 A10 L5 A11 | A14 A7 L7 A6 L6 | L6 A15 L7 A14
extrude "Extrusion18" cut sketch "Sketch14" along normal mid plane 35 contours A9 A0 | A12 A3 | A10 A4 | A14 A7
sketch "Sketch16" plane through (0, 0, 35) normal (0, 0, 1) x (1, 0, 0)
  line L0 (16.4475, 0) -> (9.185, 0) projected
  line L1 (9.185, 0) -> (9.185, -10) projected
  line L2 (9.185, -10) -> (11.3724, -10) projected
  arc A0 (11.3724, -10) -> (39.6566, -10) centre (25.5145, -5) ccw projected
  line L3 (39.6566, -10) -> (41.8442, -10) projected
  line L4 (41.8442, -10) -> (41.8442, 0) projected
  line L5 (41.8442, 0) -> (34.5815, 0) projected
  line L6 (34.5815, 0) -> (34.5815, -5) projected
  arc A1 (16.4475, -5) -> (34.5815, -5) centre (25.5145, -5) ccw projected
  line L7 (16.4475, -5) -> (16.4475, 0) projected
  arc A2 (13.0145, -12.5) -> (38.0145, -12.5) centre (25.5145, -12.5) ccw
  line L8 (16.4475, 0) -> (34.5815, 0)
  line L9 (25.5145, -5) -> (25.5145, -20)
  arc A3 (11.3724, -10) -> (39.6566, -10) centre (25.5145, -5) ccw projected
  line L10 (13.0145, -13.2916) -> (13.0145, 0)
  line L11 (38.0145, -13.2916) -> (38.0145, 0)
  line L12 (16.4475, 0) -> (9.185, 0) projected
  line L13 (41.8442, 0) -> (34.5815, 0) projected
  point P0 (0, 0)
  dimension "d205" = 25
  constraints: 8 end point, 6 point on circle, 4 point on line, 3 tangent, 2 perpendicular, 2 vertical, 1 centre point, 1 horizontal
  measures "d205" diameter of A2
extrude "Extrusion19" add sketch "Sketch16" along normal blind 17 contours L7 A1 L9 A0 A2 L10 L0 | L8 L6 A1 L7 | L5 L11 A2 A0 L9 A1 L6 | A0 A2
sketch "Sketch17" plane through (0, 0, 52) normal (0, 0, 1) x (1, 0, 0)
  line L0 (38.0145, 0) -> (13.0145, 0) projected
  line L1 (13.0145, 0) -> (13.0145, -12.5) projected
  arc A0 (13.0145, -12.5) -> (38.0145, -12.5) centre (25.5145, -12.5) ccw projected
  line L2 (38.0145, -12.5) -> (38.0145, 0) projected
  circle A1 centre (25.5145, -12.5) radius 5
  point P0 (0, 0)
  dimension "d208" = 10
  constraints: 1 centre point, 1 coincident
  measures "d208" diameter of A1
extrude "Extrusion20" cut sketch "Sketch17" against normal blind 17 contours A1
sketch "Sketch18" plane through (0, 0, 35) normal (0, 0, -1) x (-1, 0, 0)
  circle A0 centre (-25.5145, -12.5) radius 5 projected
  line L0 (-38.0145, 0) -> (-13.0145, 0) projected
  line L1 (-13.0145, 0) -> (-13.0145, -12.5) projected
  arc A1 (-38.0145, -12.5) -> (-13.0145, -12.5) centre (-25.5145, -12.5) ccw projected
  line L2 (-38.0145, -12.5) -> (-38.0145, 0) projected
  line L3 (-25.5145, -20.8716) -> (-32.7645, -16.6858)
  line L4 (-32.7645, -16.6858) -> (-32.7645, -8.3142)
  line L5 (-32.7645, -8.3142) -> (-25.5145, -4.1284)
  line L6 (-25.5145, -4.1284) -> (-18.2645, -8.3142)
  line L7 (-18.2645, -8.3142) -> (-18.2645, -16.6858)
  line L8 (-18.2645, -16.6858) -> (-25.5145, -20.8716)
  line L9 (-32.7645, -8.3142) -> (-32.7645, 0)
  line L10 (-18.2645, -8.3142) -> (-18.2645, 0)
  point P0 (0, 0)
  dimension "d224" = 14.5
  constraints: 16 end point, 2 point on line, 1 coincident, 1 parallel, 1 perpendicular, 13 other
  measures "d224" distance between parallel lines of L3 L6
extrude "Extrusion21" cut sketch "Sketch18" against normal blind 9 contours L0 L10 L6 L5 L9 | L5 L6 L7 L8 L3 L4
sketch "Sketch19" plane through (0, 0, 52) normal (0, 0, 1) x (1, 0, 0)
  circle A0 centre (25.5145, -12.5) radius 5 projected
  line L0 (38.0145, 0) -> (13.0145, 0) projected
  line L1 (13.0145, 0) -> (13.0145, -12.5) projected
  arc A1 (13.0145, -12.5) -> (38.0145, -12.5) centre (25.5145, -12.5) ccw projected
  line L2 (38.0145, -12.5) -> (38.0145, 0) projected
  circle A2 centre (25.5145, -12.5) radius 4.75
  point P0 (0, 0)
  dimension "d214" = 9.5
  constraints: 1 centre point, 1 coincident
  measures "d214" diameter of A2
extrude "Extrusion22" add sketch "Sketch19" against normal up to surface (8 mm away) contours A0
sketch "Sketch20" plane through (34.5815, 0, 0) normal (0, 1, 0) x (1, 0, 0)
  line L0 (-18.134, 0) -> (-18.134, -35) projected
  line L1 (-25.3965, 0) -> (-18.134, 0) projected
  line L2 (-25.3965, 0) -> (-25.3965, -11.668) projected
  line L3 (-25.3965, -11.668) -> (-22.7245, -11.668) projected
  line L4 (-22.7245, -11.668) -> (-22.7245, -23.332) projected
  line L5 (-22.7245, -23.332) -> (-25.3965, -23.332) projected
  line L6 (-25.3965, -23.332) -> (-25.3965, -35) projected
  line L7 (-21.567, -35) -> (-25.3965, -35) projected
  line L8 (-21.567, -35) -> (-21.567, -52) projected
  line L9 (3.433, -52) -> (-21.567, -52) projected
  line L10 (3.433, -35) -> (3.433, -52) projected
  line L11 (7.2627, -35) -> (3.433, -35) projected
  line L12 (7.2627, -35) -> (7.2627, -23.332) projected
  line L13 (7.2627, -23.332) -> (4.5905, -23.332) projected
  line L14 (4.5905, -23.332) -> (4.5905, -11.668) projected
  line L15 (4.5905, -11.668) -> (7.2627, -11.668) projected
  line L16 (7.2627, -11.668) -> (7.2627, 0) projected
  line L17 (0, 0) -> (7.2627, 0) projected
  line L18 (0, 0) -> (0, -35) projected
  line L19 (-1.817, -35) -> (-1.817, -44) projected
  line L20 (-1.817, -44) -> (-16.317, -44) projected
  line L21 (-16.317, -44) -> (-16.317, -35) projected
  circle A0 centre (-21.8965, -5.833) radius 1.5 projected
  circle A1 centre (-21.8965, -29.167) radius 1.5 projected
  circle A2 centre (3.7625, -29.167) radius 1.5 projected
  circle A3 centre (3.7625, -5.833) radius 1.5 projected
  line L22 (7.2627, -23.332) -> (7.2627, -35) projected
  line L23 (7.2627, -23.532) -> (4.2905, -23.532)
  line L24 (4.2905, -23.532) -> (4.2905, -11.468)
  line L25 (4.2905, -11.468) -> (7.2627, -11.468)
  line L26 (7.2627, -11.468) -> (7.2627, -23.532)
  line L27 (-25.3965, -29.167) -> (-25.3965, -23.332) projected
  line L28 (-25.3965, -23.532) -> (-22.4245, -23.532)
  line L29 (-22.4245, -23.532) -> (-22.4245, -11.468)
  line L30 (-22.4245, -11.468) -> (-25.3965, -11.468)
  line L31 (-25.3965, -11.468) -> (-25.3965, -23.532)
  line L32 (-16.317, -35) -> (-18.134, -35) projected
  line L33 (0, -35) -> (-1.817, -35) projected
  point P0 (-34.5815, 0)
  dimension "d217" = 0.2
  dimension "d218" = 0.2
  dimension "d219" = 0.2
  dimension "d220" = 0.3
  dimension "d221" = 0.3
  constraints: 16 end point, 4 parallel, 3 point on line, 2 horizontal, 2 perpendicular
  measures "d217" distance between parallel lines of L5 L28
  measures "d218" distance between parallel lines of L3 L30
  measures "d219" distance between parallel lines of L13 L23
  measures "d220" distance between parallel lines of L4 L29
  measures "d221" distance between parallel lines of L14 L24
extrude "Extrusion23" cut sketch "Sketch20" against normal blind 27.5 contours L30 L29 L28 L6 L5 L4 L3 L2 | L3 L4 L5 L31 | L16 L15 L14 L13 L12 L23 L24 L25 | L26 L13 L14 L15
equation "\"d59\" = 0.5 * d58"
equation "\"d60\" = d59"
equation "\"d63\" = d59"
equation "\"d64\" = d60"
equation "\"d72\" = d71"
equation "\"d73\" = d71"
equation "\"d74\" = d72"
equation "\"d76\" = d75"
equation "\"d77\" = d75"
equation "\"d78\" = d75"
equation "\"d85\" = 0.5 * d84"
equation "\"d110\" = d108"
equation "\"d111\" = d108"
equation "\"d112\" = d108"
equation "\"d113\" = d108"
equation "\"d114\" = d108"
equation "\"d115\" = d108"
equation "\"d117\" = d116"
equation "\"d118\" = d116"
equation "\"d119\" = d116"
equation "\"d120\" = d116"
equation "\"d121\" = d116"
equation "\"d122\" = d116"
equation "\"d131\" = 0.5 * d130"
equation "\"d132\" = 0.5 * d129"
equation "\"d133\" = 0.5 * d129"
equation "\"d134\" = 0.25 * d130"
equation "\"d135\" = d134"
equation "\"d54\" = 0.5 * d53"
equation "\"d57\" = d54"
equation "\"d53\" = 5.843"
body "Solid1"
